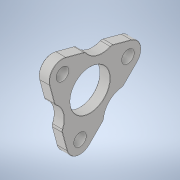
# Autodesk Inventor part: Torque_Triangle
Saved by Autodesk Inventor 2021 (Build 250183000, 183)
## iProperties
Created: 2020-10-13
Part Number: Torque_Triangle
Material: Generic
Document SubType Name: Modeling
Designer: PhotonUser
Density: 1 g/cm^3
Appearance: Default
Author: PhotonUser
Autodesk Inventor part; units mm, degrees
ref_plane "YZ Plane" through (0, 0, 0) normal (1, 0, 0) x (0, 1, 0)
ref_plane "XZ Plane" through (0, 0, 0) normal (0, 1, 0) x (-1, 0, 0)
ref_plane "XY Plane" through (0, 0, 0) normal (0, 0, 1) x (1, 0, 0)
sketch "Sketch1" plane through (0, 0, 0) normal (1, 0, 0) x (0, 1, 0)
  circle A0 centre (8.0564, -30.067) radius 5.0038
  circle A1 centre (22.0106, 22.0106) radius 5.0038
  circle A2 centre (-30.067, 8.0564) radius 5.0038
  circle A3 centre (8.0564, -30.067) radius 10.4775
  circle A4 centre (22.0106, 22.0106) radius 10.4775
  circle A5 centre (-30.067, 8.0564) radius 10.4775
  circle A6 centre (0, 0) radius 15.875
  circle A7 centre (30.067, -8.0564) radius 5.0038
  circle A8 centre (-22.0106, -22.0106) radius 5.0038
  circle A9 centre (-8.0564, 30.067) radius 5.0038
  line L0 (32.1311, 19.2988) -> (18.1769, -32.7788)
  line L1 (0.6477, -37.4758) -> (-37.4758, 0.6477)
  line L2 (-32.7788, 18.1769) -> (19.2988, 32.1311)
  dimension "d0" = 20.955
  dimension "d1" = 20.955
  dimension "d2" = 20.955
  dimension "d3" = 31.75
  constraints: 10 centre point, 6 end point, 6 point on circle, 6 tangent, 3 coincident
  measures "d0" diameter of A3
  measures "d1" diameter of A4
  measures "d2" diameter of A5
  measures "d3" diameter of A6
extrude "Extrusion1" add sketch "Sketch1" along normal blind 8.255 contours A3 | A3 L1 A5 L2 A4 L0 | A5 | A4
sketch "Sketch2" plane through (8.255, 0, 0) normal (1, 0, 0) x (0, 0, -1)
  line L0 (0, 0) -> (34.3386, -34.3386)
  line L1 (0, 0) -> (48.5621, 0) construction
  circle A0 centre (26.67, -26.67) radius 15.875
  circle A1 centre (9.7619, 36.4319) radius 15.875
  circle A2 centre (-36.4319, -9.7619) radius 15.875
  dimension "d6" = 45
  dimension "d7" = 31.75
  dimension "d8" = 26.67
  dimension "d11" = 360
  constraints: 4 end point, 3 centre point, 1 equal length, 1 horizontal, 1 point on line, 7 other
  measures "d6" angle of L0 L1
  measures "d7" diameter of A0
  measures "d8" horizontal distance of A0.centre L0.start
extrude "Extrusion2" cut sketch "Sketch2" against normal blind 8.255
fillet "Fillet1" radius 3.175 6 edges at (4.1275, 3.6496, 27.9379) (4.1275, -17.1296, 22.3701) (4.1275, -10.8083, -26.0197) (4.1275, -26.0197, -10.8083) (4.1275, 27.9379, 3.6496) (4.1275, 22.3701, -17.1296)
chamfer "Chamfer1" distance 0.254 angle 45 36 edges at (8.255, 12.0418, 30.1866) (8.255, 3.8133, 27.7953) (8.255, -5.6531, 21.0978) (8.255, -17.2001, 22.1648) (8.255, -25.5218, 20.1214) (8.255, -40.1875, 10.7682) (8.255, -32.1633, -4.6648) (8.255, -25.9781, -10.5952) (8.255, -15.4447, -15.4447) (8.255, -10.5952, -25.9781) (8.255, -4.6648, -32.1633) (8.255, 10.7682, -40.1875) (8.255, 20.1214, -25.5218) (8.255, 22.1648, -17.2001) (8.255, 21.0978, -5.6531) (8.255, 27.7953, 3.8133) (8.255, 30.1866, 12.0418) (8.255, 29.4193, 29.4193) (0, 30.1866, 12.0418) (0, 29.4193, 29.4193) (0, 12.0418, 30.1866) (0, 3.8133, 27.7953) (0, -5.6531, 21.0978) (0, -17.2001, 22.1648) (0, -25.5218, 20.1214) (0, -40.1875, 10.7682) (0, -32.1633, -4.6648) (0, -25.9781, -10.5952) (0, -15.4447, -15.4447) (0, -10.5952, -25.9781) (0, -4.6648, -32.1633) (0, 10.7682, -40.1875) (0, 20.1214, -25.5218) (0, 22.1648, -17.2001) (0, 21.0978, -5.6531) (0, 27.7953, 3.8133)
chamfer "Chamfer2" distance 0.254 angle 45 2 edges at (8.255, -15.875, 0) (0, -15.875, 0)
body "Solid1"
